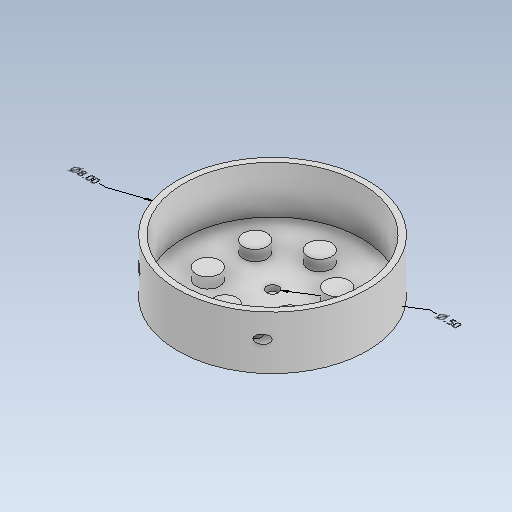
# Autodesk Inventor part: baseV01
Saved by Autodesk Inventor 2021 (Build 250183000, 183)
## iProperties
Created: 2020-05-22
Part Number: baseV01
Material: Generic
Document SubType Name: Modeling
Designer: robst
Density: 1 g/cm^3
Appearance: Default
Author: robst
Autodesk Inventor part; units mm, degrees
ref_plane "YZ Plane" through (0, 0, 0) normal (1, 0, 0) x (0, 1, 0)
ref_plane "XZ Plane" through (0, 0, 0) normal (0, 1, 0) x (-1, 0, 0)
ref_plane "XY Plane" through (0, 0, 0) normal (0, 0, 1) x (1, 0, 0)
sketch "Sketch1" plane through (0, 0, 0) normal (0, 1, 0) x (-1, 0, 0)
  circle A0 centre (0, 0) radius 101.6
  dimension "baseOutsideDiameter" = 203.2
  constraints: 1 centre point, 1 coincident
  measures "baseOutsideDiameter" diameter of A0
extrude "Extrusion1" add sketch "Sketch1" along normal blind 6.35
sketch "Sketch2" plane through (0, 6.35, 0) normal (0, 1, 0) x (1, 0, 0)
  circle A0 centre (0, 0) radius 101.6
  circle A1 centre (0, 0) radius 95.25
  dimension "d4" = 6.35
  dimension "d5" = 203.2
  constraints: 2 centre point, 2 coincident
  measures "d4" radial gap between concentric circles of A0 A1
  measures "d5" diameter of A0
extrude "Extrusion2" add sketch "Sketch2" along normal blind 50.8
sketch "Sketch3" plane through (0, 6.35, 0) normal (0, 1, 0) x (1, 0, 0)
  circle A0 centre (0, 0) radius 6.35
  dimension "wormDriveDiameer" = 12.7
  constraints: 1 centre point, 1 coincident
  measures "wormDriveDiameer" diameter of A0
extrude "Extrusion3" cut sketch "Sketch3" against normal through all
sketch "Sketch5" plane through (0, 6.35, 0) normal (0, 1, 0) x (1, 0, 0)
  circle A0 centre (0, 50.8) radius 12.7
  point P0 (0, 0)
  dimension "wormGearSupportBaseDiameter" = 25.4
  dimension "radiusOfGearSupports" = 50.8
  constraints: 1 centre point
  measures "wormGearSupportBaseDiameter" diameter of A0
  measures "radiusOfGearSupports" distance of A0.centre point (0, 0)
extrude "Extrusion5" add sketch "Sketch5" along normal blind 11.43
pattern_circular "Circular Pattern1" count 6 over 360 about axis through (0, -10, 0) along (0, 1, 0) of "Extrusion5"
sketch "Sketch6" plane through (0, 0, 0) normal (1, 0, 0) x (0, 1, 0)
  arc A0 (36.2401, 78.3957) -> (36.2401, 75.2207) centre (31.75, 76.8082) ccw projected
  circle A1 centre (31.75, 76.8082) radius 4.7625
  point P0 (0, 0)
  constraints: 1 centre point, 1 coincident, 1 concentric
extrude "Extrusion6" cut sketch "Sketch6" along normal through all both and the other way through all
equation "\"d4\" = baseThickness"
equation "\"d5\" = baseOutsideDiameter"
equation "\"baseThickness\" = 6.35"
body "Solid1"
